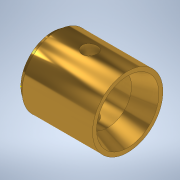
# Autodesk Inventor part: KOLBEN PART 11
Saved by Autodesk Inventor 2021 (Build 250183000, 183)
## iProperties
Created: 2020-07-03
Part Number: KOLBEN PART 11
Material: Brass, Soft Yellow
Document SubType Name: Modeling
Designer: Smit Ambardekar
Density: 8.47 g/cm^3
Appearance: Brass - Polished
Author: Smit Ambardekar
Autodesk Inventor part; units mm, degrees
ref_plane "YZ Plane" through (0, 0, 0) normal (1, 0, 0) x (0, 1, 0)
ref_plane "XY Plane" through (0, 0, 0) normal (0, 0, 1) x (1, 0, 0)
sketch "Sketch1" plane through (0, 0, 0) normal (0, 1, 0) x (-1, 0, 0)
  line L0 (0, 0) -> (0, -6.25)
  line L1 (0, 0) -> (-1, 0)
  line L2 (-1, 0) -> (-1, 0.75)
  line L3 (0, -6.25) -> (-1, -6.25)
  line L4 (-1, 0.75) -> (-15, 0.75)
  line L5 (-15, 0.75) -> (-15, -6.25)
  line L6 (-15, -6.25) -> (-1, -6.25)
  line L7 (-15, -6.25) -> (-15, -1.5)
  line L8 (-15, -6.25) -> (-15, -0.05)
  line L9 (-15, 0.75) -> (-15, -0.05)
  line L10 (-15, -0.05) -> (-11.0162, -1.5)
  line L11 (-11.0162, -1.5) -> (-4, -1.5)
  line L12 (-4, -1.5) -> (-1, -6.25)
  line L13 (-11.0162, -1.5) -> (-4, -1.5)
  dimension "d0" = 6.25
  dimension "d3" = 0.75
  dimension "d5" = 4.75
  dimension "d6" = 6.2
  dimension "d7" = 0.8
  dimension "d11" = 11
  constraints: 28 end point, 4 perpendicular, 3 horizontal, 2 point on line, 1 collinear, 1 vertical
  measures "d0" distance of L0.start L0.end
  measures "d3" distance of L1.end L2.end
  measures "d5" distance of L5.end L7.end
  measures "d6" distance of L5.end L8.end
  measures "d7" distance of L4.end L8.end
  measures "d11" distance of L7.end L11.end
revolve "Revolution1" add sketch "Sketch1" angle 360 about axis through (0, 0, -6.25) along (1, 0, 0) contours L0 L3 L12 L11 L10 L5 L4 L2 L1
sketch "Sketch2" plane through (0, 0, 0) normal (0, 0, 1) x (1, 0, 0)
  point P0 (0, 0)
ref_plane "Work Plane1" through (0, 7, 0) normal (0, 1, 0) x (-1, 0, 0)
sketch "Sketch3" plane through (0, 7, 0) normal (0, 1, 0) x (-1, 0, 0)
  line L0 (-15, -12.45) -> (-15, -0.05) projected
  line L1 (-15, -6.25) -> (-7.5, -6.25)
  circle A0 centre (-7.5, -6.25) radius 1.5
  point P0 (0, 0)
  dimension "d14" = 7.5
  dimension "d15" = 3
  constraints: 2 end point, 1 centre point, 1 coincident, 1 horizontal, 1 midpoint
  measures "d14" distance of L1.start L1.end
  measures "d15" diameter of A0
hole "Hole1" at (7.5, 7, -6.25) direction (0, -1, 0) diameter 3 end through all
body "Solid1"
